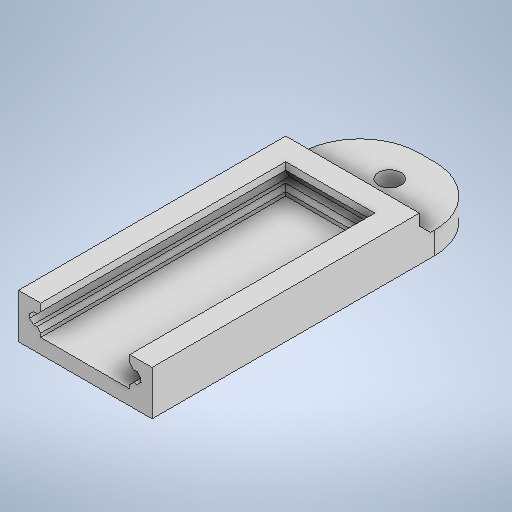
# Autodesk Inventor part: RC_Snubber
Saved by Autodesk Inventor 2025.1 (Build 291241000, 241)
## iProperties
Created: 2026-05-25
Part Number: RC_Snubber
Material: Generic
Document SubType Name: Modeling
Designer: User
Density: 1 g/cm^3
Appearance: Default
Author: User
## iProperties of the stored document RC_Snubber_3DPrint.ipt
Created: 2026-05-25
Part Number: RC_Snubber_3DPrint
Material: Generic
Document SubType Name: Modeling
Designer: User
Density: 1 g/cm^3
Appearance: Default
Author: User
Autodesk Inventor part; units mm, degrees
ref_plane "YZ Plane" through (0, 0, 0) normal (1, 0, 0) x (0, 1, 0)
ref_plane "XZ Plane" through (0, 0, 0) normal (0, 1, 0) x (-1, 0, 0)
ref_plane "XY Plane" through (0, 0, 0) normal (0, 0, 1) x (1, 0, 0)
sketch "Sketch1" plane through (0, 0, 0) normal (0, 1, 0) x (-1, 0, 0)
  line L0 (4.2628, 17.0095) -> (-9.7372, 17.0095)
  line L1 (-9.7372, 17.0095) -> (-9.7372, -14.9905)
  line L2 (-9.7372, -14.9905) -> (4.2628, -14.9905)
  line L3 (4.2628, -14.9905) -> (4.2628, 17.0095)
  line L4 (4.7628, 17.5095) -> (-10.2372, 17.5095)
  line L5 (-10.2372, 17.5095) -> (-10.2372, -15.4905)
  line L6 (-10.2372, -15.4905) -> (4.7628, -15.4905)
  line L7 (4.7628, -15.4905) -> (4.7628, 17.5095)
  point P0 (0, 0)
  dimension "d0" = 14
  dimension "d1" = 32
  dimension "d2" = 0.5
  constraints: 16 end point, 4 parallel, 2 perpendicular, 1 horizontal, 3 other
  measures "d0" distance of L2.end L1.end
  measures "d1" distance of L1.end L0.end
  measures "d2" distance between parallel lines of L3 L7
extrude "Extrusion1" add sketch "Sketch1" along normal blind 2 contours L3 L2 L1 L0 | L7 L6 L5 L4
sketch "Sketch2" plane through (0, 2, 0) normal (0, 1, 0) x (1, 0, 0)
  line L0 (-4.7628, 15.4905) -> (-4.7628, -17.5095) projected
  line L1 (10.2372, -17.5095) -> (10.2372, 15.4905) projected
  line L2 (-3.2628, 15.4905) -> (-3.2628, -17.5095)
  line L3 (8.7372, -17.5095) -> (8.7372, 15.4905)
  line L4 (-3.2628, -17.5095) -> (-6.2628, -17.5095)
  line L5 (-6.2628, -17.5095) -> (-6.2628, 15.4905)
  line L6 (-6.2628, 15.4905) -> (-3.2628, 15.4905)
  line L7 (-3.2628, 15.4905) -> (-3.2628, -17.5095)
  line L8 (8.7372, -17.5095) -> (11.7372, -17.5095)
  line L9 (11.7372, -17.5095) -> (11.7372, 15.4905)
  line L10 (11.7372, 15.4905) -> (8.7372, 15.4905)
  line L11 (8.7372, 15.4905) -> (8.7372, -17.5095)
  point P0 (0, 0)
  dimension "d5" = 1.5
  dimension "d6" = 1.5
  dimension "d7" = 3
  dimension "d8" = 3
  constraints: 20 end point, 6 parallel, 2 horizontal, 2 perpendicular, 1 point on line
  measures "d5" distance between parallel lines of L0 L2
  measures "d6" distance between parallel lines of L1 L3
  measures "d7" distance of L5.end L6.end
  measures "d8" distance of L10.end L9.end
extrude "Extrusion2" add sketch "Sketch2" along normal blind 1
sketch "Sketch3" plane through (0, 3, 0) normal (0, 1, 0) x (1, 0, 0)
  line L0 (-6.2628, 15.4905) -> (-6.2628, -17.5095) projected
  line L1 (11.7372, -17.5095) -> (11.7372, 15.4905) projected
  line L2 (-6.2628, -17.5095) -> (-4.7628, -17.5095) projected
  line L3 (-3.2628, 15.4905) -> (-6.2628, 15.4905) projected
  line L4 (-6.2628, -17.5095) -> (-4.7628, -17.5095)
  line L5 (-4.7628, -17.5095) -> (-4.7628, 15.4905)
  line L6 (-4.7628, 15.4905) -> (-6.2628, 15.4905)
  line L7 (-6.2628, 15.4905) -> (-6.2628, -17.5095)
  line L8 (10.2372, -17.5095) -> (10.2372, 15.4905) projected
  line L9 (11.7372, -17.5095) -> (10.2372, -17.5095)
  line L10 (10.2372, -17.5095) -> (10.2372, 15.4905)
  line L11 (10.2372, 15.4905) -> (11.7372, 15.4905)
  line L12 (11.7372, 15.4905) -> (11.7372, -17.5095)
  point P0 (0, 0)
  constraints: 16 end point, 4 parallel, 2 horizontal, 2 perpendicular, 1 midpoint
extrude "Extrusion3" add sketch "Sketch3" along normal blind 1.5
sketch "Sketch4" plane through (0, 4.5, 0) normal (0, 1, 0) x (1, 0, 0)
  line L0 (-4.7628, 15.4905) -> (-6.2628, 15.4905) projected
  line L1 (-6.2628, 15.4905) -> (-6.2628, -17.5095) projected
  line L2 (-6.2628, -17.5095) -> (-4.7628, -17.5095) projected
  line L3 (-4.7628, -17.5095) -> (-4.7628, 15.4905) projected
  line L4 (11.7372, -17.5095) -> (11.7372, 15.4905) projected
  line L5 (11.7372, 15.4905) -> (10.2372, 15.4905) projected
  line L6 (10.2372, 15.4905) -> (10.2372, -17.5095) projected
  line L7 (10.2372, -17.5095) -> (11.7372, -17.5095) projected
  line L8 (8.7372, 15.4905) -> (8.7372, -17.5095) projected
  line L9 (-3.2628, -17.5095) -> (-3.2628, 15.4905) projected
  line L10 (8.7372, 15.4905) -> (-3.2628, 15.4905) projected
  line L11 (-6.2628, -17.5095) -> (-3.2628, -17.5095)
  line L12 (-3.2628, -17.5095) -> (-3.2628, 15.4905)
  line L13 (-3.2628, 15.4905) -> (-6.2628, 15.4905)
  line L14 (-6.2628, 15.4905) -> (-6.2628, -17.5095)
  line L15 (11.7372, -17.5095) -> (8.7372, -17.5095)
  line L16 (8.7372, -17.5095) -> (8.7372, 15.4905)
  line L17 (8.7372, 15.4905) -> (11.7372, 15.4905)
  line L18 (11.7372, 15.4905) -> (11.7372, -17.5095)
  point P0 (0, 0)
  constraints: 16 end point, 4 parallel, 2 horizontal, 2 perpendicular
extrude "Extrusion4" add sketch "Sketch4" along normal blind 1.5
chamfer "Chamfer1" distance 0.5 angle 45 4 edges at (-3.2628, 3, 1.0095) (8.7372, 3, 1.0095) (10.2372, 3, 1.0095) (-4.7628, 3, 1.0095)
chamfer "Chamfer2" distance 0.5 angle 45 4 edges at (-4.7628, 4.5, 1.0095) (10.2372, 4.5, 1.0095) (8.7372, 4.5, 1.0095) (-3.2628, 4.5, 1.0095)
sketch "Sketch5" plane through (0, 2, 0) normal (0, -1, 0) x (1, 0, 0)
  line L0 (-4.7628, -15.4905) -> (-4.7628, 17.5095) projected
  line L1 (-6.2628, 17.5095) -> (-4.7628, 17.5095) projected
  line L2 (-6.2628, -15.4905) -> (-6.2628, 17.5095) projected
  line L3 (-4.7628, -15.4905) -> (-6.2628, -15.4905) projected
  line L4 (10.2372, 17.5095) -> (10.2372, -15.4905) projected
  line L5 (11.7372, -15.4905) -> (10.2372, -15.4905) projected
  line L6 (11.7372, 17.5095) -> (11.7372, -15.4905) projected
  line L7 (10.2372, 17.5095) -> (11.7372, 17.5095) projected
  point P0 (0, 0)
extrude "Extrusion5" add sketch "Sketch5" along normal up to surface (2 mm away)
sketch "Sketch6" plane through (11.7372, 0, -15.4905) normal (0, 0, -1) x (-1, 0, 0)
  line L0 (0, 0) -> (0, 6) projected
  line L1 (18, 0) -> (0, 0) projected
  line L2 (0, 6) -> (3, 6) projected
  line L3 (15, 6) -> (18, 6) projected
  line L4 (18, 0) -> (18, 6) projected
  line L5 (16.5, 4) -> (16, 4.5) projected
  line L6 (15.5, 4.5) -> (16, 4.5) projected
  line L7 (16.5, 3.5) -> (16.5, 4) projected
  line L8 (16, 3) -> (16.5, 3.5) projected
  line L9 (15.5, 3) -> (16, 3) projected
  line L10 (2, 3) -> (2.5, 3) projected
  line L11 (1.5, 3.5) -> (2, 3) projected
  line L12 (1.5, 3.5) -> (1.5, 4) projected
  line L13 (2, 4.5) -> (1.5, 4) projected
  line L14 (2, 4.5) -> (2.5, 4.5) projected
  line L15 (2.5, 4.5) -> (15.5, 4.5)
  line L16 (3, 2.5) -> (2.5, 3) projected
  line L17 (15, 2.5) -> (15.5, 3) projected
  line L18 (2.5, 3) -> (15.5, 3)
  line L19 (3, 5) -> (3, 6) projected
  line L20 (15, 5) -> (15, 6) projected
  line L21 (3, 6) -> (15, 6)
  point P0 (11.7372, 0)
  constraints: 6 end point, 2 horizontal, 1 parallel
extrude "Extrusion6" add sketch "Sketch6" along normal blind 1.5
sketch "Sketch7" plane through (11.7372, 0, -16.9905) normal (0, 0, -1) x (-1, 0, 0)
  line L0 (0, 6) -> (0, 0) projected
  line L1 (0, 0) -> (18, 0) projected
  line L2 (18, 6) -> (18, 0) projected
  line L3 (0, 6) -> (18, 6)
  line L4 (18, 6) -> (18, 0)
  line L5 (18, 0) -> (0, 0)
  line L6 (0, 0) -> (0, 6)
  point P0 (11.7372, 0)
  constraints: 8 end point, 2 parallel, 1 horizontal, 1 perpendicular
extrude "Extrusion7" add sketch "Sketch7" along normal blind 1.5
chamfer "Chamfer3" distance 0.5 angle 45 2 edges at (2.7372, 3, -15.4905) (2.7372, 4.5, -15.4905)
sketch "Sketch8" plane through (11.7372, 0, -18.4905) normal (0, 0, -1) x (-1, 0, 0)
  line L0 (0, 6) -> (0, 0) projected
  line L1 (0, 0) -> (18, 0) projected
  line L2 (18, 0) -> (18, 6) projected
  line L3 (18, 6) -> (0, 6) projected
  point P0 (11.7372, 0)
extrude "Extrusion8" add sketch "Sketch8" along normal blind 10
sketch "Sketch9" plane through (0, 6, 0) normal (0, 1, 0) x (1, 0, 0)
  line L0 (-6.2628, 28.4905) -> (11.7372, 28.4905) projected
  line L1 (-6.2628, -17.5095) -> (-6.2628, 28.4905) projected
  line L2 (11.7372, 28.4905) -> (-6.2628, 28.4905)
  line L3 (-6.2628, 28.4905) -> (-6.2628, 18.4905)
  line L4 (-6.2628, 18.4905) -> (11.7372, 18.4905)
  line L5 (11.7372, 18.4905) -> (11.7372, 28.4905)
  point P0 (0, 0)
  dimension "d32" = 10
  constraints: 8 end point, 2 parallel, 1 horizontal, 1 perpendicular, 1 point on line
  measures "d32" distance of L3.end L2.end
extrude "Extrusion9" cut sketch "Sketch9" against normal blind 3
sketch "Sketch10" plane through (0, 3, 0) normal (0, 1, 0) x (1, 0, 0)
  line L0 (11.7372, 28.4905) -> (11.7372, 18.4905) projected
  line L1 (-6.2628, 18.4905) -> (-6.2628, 28.4905) projected
  line L2 (11.7372, 18.4905) -> (-6.2628, 18.4905) projected
  line L3 (11.7372, 28.4905) -> (-6.2628, 18.4905)
  circle A0 centre (2.7372, 23.4905) radius 1.5
  point P0 (0, 0)
  dimension "d35" = 3
  constraints: 2 end point, 1 centre point, 1 midpoint
  measures "d35" diameter of A0
extrude "Extrusion10" cut sketch "Sketch10" against normal blind 3 contours A0 L3 | L3 A0
fillet "Fillet1" radius 8 2 edges at (-6.2628, 1.5, -28.4905) (11.7372, 1.5, -28.4905)
chamfer "Chamfer4" distance 1.5 angle 45 1 edges at (2.7372, 3, -18.4905)
body "Solid1"
